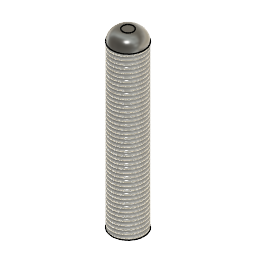
Tower Holder (Autodesk Fusion 360 design; units mm, degrees)
part number: 2026-02-19-12-58-25-626
Autodesk Fusion 360 part; units mm, degrees
sketch "Sketch1" plane through (0, 0, 0) normal (0, 0, 1) x (1, 0, 0)
  circle A0 centre (0, 0) radius 15
  dimension "d1" = 30
  constraint coincident A0.centre origin
  measures "d1" diameter of A0
extrude "Extrude1" add sketch "Sketch1" along normal blind 160
thread "Thread1" "ISO Metric profile 30.0 M30x3.5 M30x3.5 6g" major diameter 29.7345 minor diameter 25.732 pitch 3.5 angle 60 resizes the face on face at (14.9814, -0.7477, 106.6667)
fillet "Fillet1" radius 10 1 faces at (-1.5399, 1.0022, 160)
